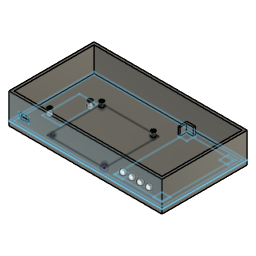
espOsmo (Autodesk Fusion 360 design; units mm, degrees)
Autodesk Fusion 360 part; units mm, degrees
sketch "ESP32 Devkit Board" plane through (0, 0, 0) normal (0, 0, 1) x (1, 0, 0)
  line L0 (0, 0) -> (-66, 0)
  line L1 (-66, 0) -> (-66, 63)
  line L2 (-66, 63) -> (0, 63)
  line L3 (0, 63) -> (0, 0)
  circle A0 centre (-63, 60) radius 1.5
  circle A1 centre (-3, 60) radius 1.5
  circle A2 centre (-3, 3) radius 1.5
  circle A3 centre (-63, 3) radius 1.5
  line L4 (-67.9, 17) -> (-89, 17)
  line L5 (-89, 17) -> (-89, 60)
  line L6 (-89, 60) -> (-67.9, 60)
  line L7 (-67.9, 60) -> (-67.9, 17)
  circle A4 centre (-70.4, 54) radius 1.5
  circle A5 centre (-86.5, 23) radius 1.5
  line L8 (13, 0) -> (67, 0)
  line L9 (67, 0) -> (67, 82.5)
  line L10 (67, 82.5) -> (13, 82.5)
  line L11 (13, 82.5) -> (13, 0)
  line L12 (-100, -5) -> (72, -5)
  line L13 (72, -5) -> (72, 88)
  line L14 (72, 88) -> (-100, 88)
  line L15 (-100, 88) -> (-100, -5)
  line L16 (12, -1) -> (22, -1)
  line L17 (22, -1) -> (22, 9)
  line L18 (22, 9) -> (12, 9)
  line L19 (12, 9) -> (12, -1)
  line L20 (68, -1) -> (58, -1)
  line L21 (58, -1) -> (58, 9)
  line L22 (58, 9) -> (68, 9)
  line L23 (68, 9) -> (68, -1)
  line L24 (69, 85) -> (59, 85)
  line L25 (59, 85) -> (59, 75)
  line L26 (59, 75) -> (69, 75)
  line L27 (69, 75) -> (69, 85)
  line L28 (11, 85) -> (21, 85)
  line L29 (21, 85) -> (21, 75)
  line L30 (21, 75) -> (11, 75)
  line L31 (11, 75) -> (11, 85)
  line L32 (-103, 91) -> (75, 91)
  line L33 (75, 91) -> (75, -8)
  line L34 (75, -8) -> (-103, -8)
  line L35 (-103, -8) -> (-103, 91)
  dimension "d1" = 66
  dimension "d2" = 63
  dimension "d3" = 3
  dimension "d4" = 3
  dimension "d5" = 3
  dimension "d6" = 3
  dimension "d7" = 3
  dimension "d8" = 3
  dimension "d9" = 3
  dimension "d10" = 3
  dimension "d11" = 3
  dimension "d12" = 3
  dimension "d13" = 3
  dimension "d14" = 3
  dimension "d15" = 21.1
  dimension "d16" = 43
  dimension "d17" = 3
  dimension "d18" = 6
  dimension "d19" = 2.5
  dimension "d20" = 3
  dimension "d21" = 2.5
  dimension "d22" = 6
  dimension "d23" = 54
  dimension "d24" = 82.5
  dimension "d69" = 10
  dimension "d70" = 10
  dimension "d71" = 10
  dimension "d72" = 10
  dimension "d73" = 10
  dimension "d74" = 10
  dimension "d75" = 10
  dimension "d76" = 10
  constraint horizontal L0
  constraint vertical L1
  constraint horizontal L2
  constraint vertical L3
  constraint coincident L0.start L3.end
  constraint horizontal L4
  constraint vertical L5
  constraint horizontal L6
  constraint vertical L7
  constraint horizontal L8
  constraint vertical L9
  constraint horizontal L10
  constraint vertical L11
  constraint horizontal L12
  constraint vertical L13
  constraint horizontal L14
  constraint vertical L15
  constraint horizontal L16
  constraint vertical L17
  constraint horizontal L18
  constraint vertical L19
  constraint horizontal L20
  constraint vertical L21
  constraint horizontal L22
  constraint vertical L23
  constraint horizontal L24
  constraint vertical L25
  constraint horizontal L26
  constraint vertical L27
  constraint horizontal L28
  constraint vertical L29
  constraint horizontal L30
  constraint vertical L31
  constraint horizontal L32
  constraint vertical L33
  constraint horizontal L34
  constraint vertical L35
  measures "d1" distance of L0.start L0.end
  measures "d2" distance of L0.start L2.end
  measures "d3" diameter of A0
  measures "d4" distance of L2 A0.centre
  measures "d5" distance of L1 A0.centre
  measures "d6" diameter of A1
  measures "d7" distance of L2 A1.centre
  measures "d8" distance of L3 A1.centre
  measures "d9" diameter of A2
  measures "d10" distance of L0 A2.centre
  measures "d11" distance of L3 A2.centre
  measures "d12" diameter of A3
  measures "d13" distance of L1 A3.centre
  measures "d14" distance of L0 A3.centre
  measures "d15" distance of L4.start L4.end
  measures "d16" distance of L4.start L6.end
  measures "d17" diameter of A4
  measures "d18" distance of L6 A4.centre
  measures "d19" distance of L7 A4.centre
  measures "d20" diameter of A5
  measures "d21" distance of L5 A5.centre
  measures "d22" distance of L4 A5.centre
  measures "d23" distance of L8.start L8.end
  measures "d24" distance of L8.start L10.end
  measures "d69" distance of L16.start L16.end
  measures "d70" distance of L16.start L18.end
  measures "d71" distance of L20.start L20.end
  measures "d72" distance of L20.start L22.end
  measures "d73" distance of L24.start L24.end
  measures "d74" distance of L24.start L26.end
  measures "d75" distance of L28.start L28.end
  measures "d76" distance of L28.start L30.end
extrude "Extrude1" add sketch "ESP32 Devkit Board" along normal blind 1 contours L0 L1 L2 L3 | A0 | A1 | A2 | A3 | L4 L5 L6 L7 | A4 | A5 | L8 L11 L17 L18 | L8 L11 L16 L17 L18 L19 | L8 L9 L10 L11 L17 L18 L21 L22 L25 L26 L29 L30 | L8 L9 L21 L22 | L8 L9 L20 L21 L22 L23 | L10 L11 L28 L29 L30 L31 | L10 L11 L29 L30 | L9 L10 L25 L26 | L9 L10 L24 L25 L26 L27 | L12 L13 L14 L15 makes body 1
extrude "Extrude2" add sketch "ESP32 Devkit Board" along normal blind 6 separate body contours A4 makes body 2
extrude "Extrude3" add sketch "ESP32 Devkit Board" along normal blind 6 separate body contours A5 makes body 3
extrude "Extrude4" add sketch "ESP32 Devkit Board" along normal blind 6 separate body contours A0 | A1 | A2 | A3 makes body 4 at (-4.3173, 60.7174, 4) makes body 5 at (-1.5019, 2.9252, 4) makes body 6 at (-61.7201, 60.7822, 4) makes body 7 at (-62.5937, 4.4439, 4)
move_face "OffsetFaces1" offset 1 1 faces at (-85.5075, 24.1247, 4) on bodies 3
move_face "OffsetFaces2" offset 1 1 faces at (-62.5937, 4.4439, 4) on bodies 7
move_face "OffsetFaces3" offset 1 1 faces at (-69.4075, 55.1247, 4) on bodies 2
move_face "OffsetFaces4" offset 1 1 faces at (-61.7201, 60.7822, 4) on bodies 6
move_face "OffsetFaces5" offset 1 1 faces at (-4.3173, 60.7174, 4) on bodies 4
move_face "OffsetFaces6" offset 1 1 faces at (-1.5019, 2.9252, 4) on bodies 5
hole "Hole1" at (-63, 60, 0) direction (0, 0, 1) diameter 2.529 depth 16 tip angle 118 bodies 1 6
thread "Thread1" "ISO Metric profile 3.0 M3x0.5 M3x0.5 6H" major diameter 3.086 minor diameter 2.529 pitch 0.5 angle 60 modelled right hand crest width 0.1368 on face at (-62.1872, 59.0313, 2) crest through (-64.2645, 60, 0.125) on face at (-62.2365, 58.992, 0.3333) crest through (-64.2645, 60, 0.125) on bodies 1 6
hole "Hole2" at (-3, 60, 0) direction (0, 0, 1) diameter 2.529 depth 16 tip angle 118 bodies 1 4
thread "Thread2" "ISO Metric profile 3.0 M3x0.5 M3x0.5 6H" major diameter 3.086 minor diameter 2.529 pitch 0.5 angle 60 modelled right hand crest width 0.1368 on face at (-4.2641, 59.9685, 0.3333) crest through (-4.2645, 60, 0.125) on face at (-4.2641, 60.0315, 2) crest through (-4.2645, 60, 0.125) on bodies 1 4
hole "Hole3" at (-86.5, 23, 0) direction (0, 0, 1) diameter 2.529 depth 29 tip angle 118 bodies 1 3
thread "Thread3" "ISO Metric profile 3.0 M3x0.5 M3x0.5 6H" major diameter 3.086 minor diameter 2.529 pitch 0.5 angle 60 modelled right hand crest width 0.1368 on face at (-86.9912, 24.1652, 2) crest through (-87.7645, 23, 0.125) on face at (-86.9912, 24.1652, 0.3333) crest through (-87.7645, 23, 0.125) on bodies 1 3
hole "Hole4" at (-70.4, 54, 0) direction (0, 0, 1) diameter 2.529 depth 29 tip angle 118 bodies 1 2
thread "Thread4" "ISO Metric profile 3.0 M3x0.5 M3x0.5 6H" major diameter 3.086 minor diameter 2.529 pitch 0.5 angle 60 modelled right hand crest width 0.1368 on face at (-69.9088, 52.8348, 0.3333) crest through (-71.6645, 54, 0.125) on face at (-69.9675, 52.8118, 2) crest through (-71.6645, 54, 0.125) on bodies 1 2
hole "Hole5" at (-3, 3, 0) direction (0, 0, 1) diameter 2.529 depth 29 tip angle 118 bodies 1 5
thread "Thread5" "ISO Metric profile 3.0 M3x0.5 M3x0.5 6H" major diameter 3.086 minor diameter 2.529 pitch 0.5 angle 60 modelled right hand crest width 0.1368 on face at (-2.937, 4.2629, 2) crest through (-4.2645, 3, 0.125) on face at (-2.8741, 4.2582, 0.6667) crest through (-4.2645, 3, 0.125) on bodies 1 5
hole "Hole6" at (-63, 3, 0) direction (0, 0, 1) diameter 2.529 depth 29 tip angle 118 bodies 1 7
thread "Thread6" "ISO Metric profile 3.0 M3x0.5 M3x0.5 6H" major diameter 3.086 minor diameter 2.529 pitch 0.5 angle 60 modelled right hand crest width 0.1368 on face at (-62.8741, 4.2582, 0.6667) crest through (-64.2645, 3, 0.125) on face at (-62.8741, 1.7418, 2) crest through (-64.2645, 3, 0.125) on bodies 1 7
extrude "Extrude5" add sketch "ESP32 Devkit Board" along normal blind 10 separate body contours L8 L11 L16 L17 L18 L19 | L8 L9 L20 L21 L22 L23 | L10 L11 L28 L29 L30 L31 | L9 L10 L24 L25 L26 L27 makes body 8 at (65.6667, 85, 3.3333) makes body 9 at (15.3333, -1, 3.3333) makes body 10 at (68, 5.6667, 3.3333) makes body 11 at (11, 78.3333, 3.3333)
extrude "Extrude6" add sketch "ESP32 Devkit Board" along normal blind 30 contours L32 L33 L34 L35 bodies 1
sketch "Sketch2" plane through (0, -8, 0) normal (0, -1, 0) x (1, 0, 0)
  line L0 (-103, 0) -> (75, 0)
  line L1 (75, 0) -> (75, 30)
  line L2 (75, 30) -> (-103, 30)
  line L3 (-103, 30) -> (-103, 0)
  circle A0 centre (60, 15) radius 1.4142
  circle A1 centre (50, 15) radius 1
  circle A2 centre (40, 15) radius 1.4923
  circle A3 centre (30, 15) radius 1.4142
  line L4 (-91, 15) -> (-80, 15)
  line L5 (-80, 15) -> (-80, 9)
  line L6 (-80, 9) -> (-91, 9)
  line L7 (-91, 9) -> (-91, 15)
  dimension "d81" = 11
  dimension "d82" = 6
  constraint horizontal L4
  constraint vertical L5
  constraint horizontal L6
  constraint vertical L7
  measures "d81" distance of L4.start L4.end
  measures "d82" distance of L4.start L6.end
hole "Hole7" at (30, -8, 15) at (40, -8, 15) at (50, -8, 15) at (60, -8, 15) direction (0, 1, 0) diameter 3.8 depth 3 tip angle 118 bodies 1
extrude "Extrude7" cut sketch "Sketch2" against normal blind 9 contours L4 L5 L6 L7 bodies 1
extrude "Extrude8" add sketch "ESP32 Devkit Board" against normal blind 5 contours L0 L1 L2 L3 | A0 | A1 | A2 | A3 | L4 L5 L6 L7 | A4 | A5 | L8 L11 L17 L18 | L8 L11 L16 L17 L18 L19 | L8 L9 L10 L11 L17 L18 L21 L22 L25 L26 L29 L30 | L8 L9 L21 L22 | L8 L9 L20 L21 L22 L23 | L10 L11 L28 L29 L30 L31 | L10 L11 L29 L30 | L9 L10 L25 L26 | L9 L10 L24 L25 L26 L27 | L12 L13 L14 L15 | L32 L33 L34 L35 bodies 1 2 3 4 5 6 7 8 9 10 11
